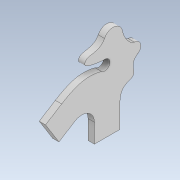
# Autodesk Inventor part: lamina_trasero
Saved by Autodesk Inventor 2021 (Build 250183000, 183)
## iProperties
Created: 2021-04-09
Part Number: lamina_trasero
Material: Genérico
Document SubType Name: Modeling
Designer: j2seb
Density: 1 g/cm^3
Appearance: Valor por defecto
Author: j2seb
Autodesk Inventor part; units mm, degrees
ref_plane "YZ Plane" through (0, 0, 0) normal (1, 0, 0) x (0, 1, 0)
ref_plane "XZ Plane" through (0, 0, 0) normal (0, 1, 0) x (-1, 0, 0)
ref_plane "XY Plane" through (0, 0, 0) normal (0, 0, 1) x (1, 0, 0)
sketch "Boceto1" plane through (0, 0, 0) normal (1, 0, 0) x (0, 1, 0)
  line L0 (525, 5.254) -> (525, 25.254)
  line L1 (525, 25.254) -> (540, 25.254)
  arc A0 (540, 25.254) -> (548.4852, 40.5618) centre (540, 35.2596) ccw
  line L2 (548.4852, 40.5618) -> (540.5364, 53.2825)
  line L3 (540.5364, 53.2825) -> (557.4974, 63.8809)
  line L4 (557.4974, 63.8809) -> (565.4462, 51.1602)
  line L5 (525, 15.254) -> (575, 17.0001) construction
  line L6 (549.0169, 58.5817) -> (575, 17.0001) construction
  line L7 (525, 5.254) -> (540, 5.254)
  circle A1 centre (575, 17.0001) radius 4
  line L8 (565.4462, 51.1602) -> (573.8002, 37.7909) construction
  line L9 (573.8755, 23.7788) -> (571.0024, 16.8605) construction
  spline S0 degree 4 poles (565.4462, 51.1602) (573.8002, 37.7909) (573.8755, 31.3158) (573.8755, 23.7788) (571.0024, 16.8605) knots 1 1 1 1 1 2 2 2 2 2
  line L10 (578.9765, 17.4327) -> (578.7688, 19.3424) construction
  line L11 (578.7688, 19.3424) -> (580.8115, 30.4088) construction
  line L12 (580.8115, 30.4088) -> (581.5561, 33.9943) construction
  line L13 (581.5561, 33.9943) -> (588.3082, 32.4831) construction
  line L14 (588.3082, 32.4831) -> (587.0334, 24.49) construction
  line L15 (587.0334, 24.49) -> (590.1956, 18.7656) construction
  line L16 (546.3222, 5.254) -> (540, 5.254) construction
  line L17 (573.8002, 37.7909) -> (573.8755, 31.3158) construction
  line L18 (573.8755, 31.3158) -> (573.8755, 23.7788) construction
  arc A2 (591.5375, 3.1103) -> (593.375, 17.2458) centre (590.1405, 10.4791) ccw
  arc A3 (569.6718, -8.8556) -> (579.02, -6.402) centre (574.02, -6.3872) ccw
  arc A4 (555.1918, -3.2238) -> (560.0425, -5.8618) centre (559, -2) ccw
  spline S1 degree 4 poles (578.9765, 17.4327) (578.7688, 19.3424) (580.8115, 30.4088) (581.5561, 33.9943) (588.3082, 32.4831) (587.0334, 24.49) (590.1956, 18.7656) (593.375, 17.2458) knots 0 0 0 0 0 1 2 3 4 4 4 4 4
  line L19 (590.1956, 18.7656) -> (593.375, 17.2458) construction
  spline S2 degree 4 poles (555.1918, -3.2238) (553.3097, 2.6327) (551.1077, 4.616) (546.3222, 5.254) (540, 5.254) knots 0 0 0 0 0 1 1 1 1 1
  line L20 (555.1918, -3.2238) -> (553.3097, 2.6327) construction
  line L21 (553.3097, 2.6327) -> (551.1077, 4.616) construction
  line L22 (551.1077, 4.616) -> (546.3222, 5.254) construction
  line L23 (569.6718, -8.8556) -> (566.9184, -4.0055) construction
  line L24 (566.9184, -4.0055) -> (560.0425, -5.8618) construction
  spline S3 degree 2 poles (569.6718, -8.8556) (566.9184, -4.0055) (560.0425, -5.8618) knots 1 1 1 2 2 2
  line L25 (575, 17.0001) -> (525, 17.0001) construction
  line L26 (591.5375, 3.1103) -> (584.136, 1.7072) construction
  line L27 (584.136, 1.7072) -> (579.0273, -3.9321) construction
  line L28 (579.0273, -3.9321) -> (579.02, -6.402) construction
  spline S4 degree 3 poles (591.5375, 3.1103) (584.136, 1.7072) (579.0273, -3.9321) (579.02, -6.402) knots 1 1 1 1 2 2 2 2
  point P0 (0, 0)
  point P1 (571.978, 19.6207)
  dimension "d3" = 8
  dimension "d0" = 20
  dimension "d1" = 60
  dimension "d2" = 15
  dimension "d4" = 15
  dimension "d5" = 10
  dimension "d6" = 8
  dimension "d7" = 2
  dimension "d8" = 50
  constraints: 18 end point, 8 point on circle, 4 centre point, 4 coincident, 4 equal length, 3 horizontal, 2 midpoint, 2 parallel, 2 perpendicular, 2 point on line, 2 tangent, 1 vertical, 26 other
  measures "d0" distance of L7.start L0.end
  measures "d1" angle of L5 L6
  measures "d2" distance of L7.start L16.end
  measures "d4" diameter of A2
  measures "d5" diameter of A3
  measures "d6" diameter of A4
  measures "d7" angle of L5 L25
  measures "d8" distance from line of L0 point (575, 17)
extrude "Extrusión1" add sketch "Boceto1" along normal mid plane 5 contours L0 L1 A0 L2 L3 L4 S0 A1 S1 A2 S4 A3 S3 A4 S2 L7
